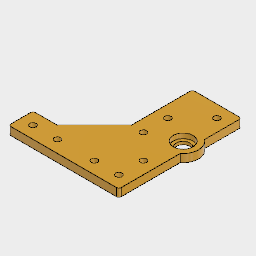
cb_epl (Autodesk Fusion 360 design; units mm, degrees)
Autodesk Fusion 360 part; units mm, degrees
sketch "Sketch1" plane through (0, 0, 0) normal (0, 0, 1) x (1, 0, 0)
  line L0 (410, 40) -> (450, 40.0001)
  line L1 (410, 40) -> (450, 40.0001)
  circle A0 centre (420.0003, -50) radius 2.51
  circle A1 centre (440.0003, -50) radius 2.51
  line L2 (450.0001, -9.6745) -> (450, 40.0001)
  line L3 (500.0003, -59.9997) -> (500.0002, -39.9997)
  line L4 (500.0002, -39.9997) -> (480.3255, -39.9998)
  circle A2 centre (490.0003, -49.9998) radius 2.51
  line L5 (410.0001, 9.9242) -> (410, 40)
  circle A3 centre (440.0001, -9.9999) radius 2.51
  circle A4 centre (420, -30) radius 2.51
  circle A5 centre (420, 30) radius 2.51
  circle A6 centre (417.6001, 0) radius 5.5
  circle A7 centre (440.0001, 10.0001) radius 2.51
  line L6 (410.0003, -60) -> (410.0001, -9.9242)
  line L7 (450.0001, -9.6745) -> (480.3255, -39.9998)
  line L8 (410.0003, -60) -> (500.0003, -59.9997)
  arc A8 (410.0001, 9.9242) -> (410.0001, -9.9242) centre (417.6001, 0) ccw
  circle A9 centre (470.0003, -49.9998) radius 2.51
  dimension "d1" = 100
  dimension "d2" = 90
  dimension "d3" = 5.02
  dimension "d4" = 10
  dimension "d5" = 10
  dimension "d6" = 5.02
  dimension "d7" = 20
  dimension "d8" = 5.02
  dimension "d9" = 5.02
  dimension "d10" = 10
  dimension "d11" = 20
  dimension "d12" = 5.02
  dimension "d13" = 5.02
  dimension "d14" = 5.02
  dimension "d15" = 5.02
  dimension "d16" = 20
  dimension "d18" = 60
  dimension "d19" = 10
  dimension "d20" = 10
  dimension "d21" = 10
  dimension "d22" = 11
  dimension "d23" = 25
  dimension "d24" = 20
  dimension "d31" = 40
  dimension "d32" = 32.4
  dimension "d33" = 40
  dimension "d34" = 10
  constraint perpendicular L3 L8
  constraint perpendicular L6 L8
  constraint vertical origin
  constraint concentric A6 A8
  constraint collinear L5 L6
  constraint perpendicular L0 L2
  measures "d2" distance of origin
  measures "d3" diameter of A0
  measures "d4" distance of L8
  measures "d6" diameter of A1
  measures "d8" diameter of A2
  measures "d9" diameter of A9
  measures "d10" distance of L3
  measures "d12" diameter of A5
  measures "d13" diameter of A4
  measures "d14" diameter of A3
  measures "d15" diameter of A7
  measures "d16" distance of origin
  measures "d19" distance of L8
  measures "d21" distance of L2
  measures "d22" diameter of A6
  measures "d23" diameter of A8
  measures "d32" distance of origin L2
  measures "d33" distance of L2 L5
extrude "Extrude1" add sketch "Sketch1" along normal blind 6.5
sketch "Sketch3" plane through (0, 0, 0) normal (0, 0, -1) x (1, 0, 0)
  circle A0 centre (470.0003, 49.9998) radius 2.51
  circle A1 centre (490.0003, 49.9998) radius 2.51
  circle A2 centre (440.0003, 50) radius 2.51
  circle A3 centre (420, -30) radius 2.51
  circle A4 centre (417.6001, 0) radius 5.5
  circle A5 centre (420.0003, 50) radius 2.51
  circle A6 centre (440.0001, -10.0001) radius 2.51
  circle A7 centre (420, 30) radius 2.51
  circle A8 centre (440.0001, 9.9999) radius 2.51
  line L0 (450, -40.0001) -> (450.0001, 9.6745)
  line L1 (450.0001, 9.6745) -> (480.3255, 39.9998)
  line L2 (480.3255, 39.9998) -> (500.0002, 39.9997)
  line L3 (500.0002, 39.9997) -> (500.0003, 59.9997)
  line L4 (500.0003, 59.9997) -> (410.0003, 60)
  line L5 (410.0003, 60) -> (410.0001, 9.9242)
  arc A9 (410.0001, 9.9242) -> (410.0001, -9.9242) centre (417.6001, 0) ccw
  line L6 (410.0001, -9.9242) -> (410, -40)
  line L7 (410, -40) -> (450, -40.0001)
  circle A10 centre (417.6001, 0) radius 8.05
  dimension "d27" = 16.1
  constraint concentric A4 A10
  measures "d27" diameter of A10
extrude "Extrude2" cut sketch "Sketch3" against normal blind 4 contours A10
fillet "Fillet1" radius 2 5 edges at (500.0003, -59.9997, 3.25) (500.0002, -39.9997, 3.25) (450, 40.0001, 3.25) (410, 40, 3.25) (410.0003, -60, 3.25)
move_body "MoveBody1" bodies 1 to x (-1, 0, 0) y (0, 1, 0) z (0, 0, -1) at (880.0586, 0, 13)
move_body "MoveBody2" bodies 1 to x (1, 0, 0) y (0, 1, 0) z (0, 0, 1) at (-420, 0, 0)
